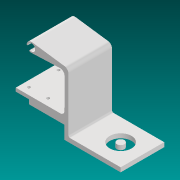
# Autodesk Inventor part: 链接板
Saved by Autodesk Inventor 2021 (Build 250183000, 183)
## iProperties
Created: 2025-04-17
Part Number: 链接板
Material: 常规
Document SubType Name: Modeling
Designer: 86155
Density: 1 g/cm^3
Appearance: 默认
Author: 86155
Autodesk Inventor part; units mm, degrees
ref_plane "YZ Plane" through (0, 0, 0) normal (1, 0, 0) x (0, 1, 0)
ref_plane "XZ Plane" through (0, 0, 0) normal (0, 1, 0) x (-1, 0, 0)
ref_plane "XY Plane" through (0, 0, 0) normal (0, 0, 1) x (1, 0, 0)
sketch "草图1" plane through (0, 0, 0) normal (0, 0, 1) x (1, 0, 0)
  circle A0 centre (0, 41) radius 4.25 projected
  circle A1 centre (0, 41) radius 4.25
  line L0 (0, 41) -> (-2.75, 36.2369)
  line L1 (0, 41) -> (5.5, 41) construction
  line L2 (0, 41) -> (-5.5, 41)
  line L3 (0.7501, 46.4486) -> (42.3728, 40.7189)
  line L4 (-15, 3) -> (-15, 6) projected
  line L5 (-15, 6) -> (-18, 6) projected
  line L6 (-18, 6) -> (-18, -8) projected
  line L7 (-4, -8) -> (-18, -8) projected
  line L8 (-4, -6) -> (-4, -8) projected
  line L9 (-4, -6) -> (4, -6) projected
  line L10 (4, -6) -> (4, -8) projected
  line L11 (18, -8) -> (4, -8) projected
  line L12 (18, 6) -> (18, -8) projected
  line L13 (18, 6) -> (15, 6) projected
  line L14 (15, 6) -> (15, 3) projected
  line L15 (15, 3) -> (13.5, 3) projected
  line L16 (13.5, 3) -> (13.5, 2) projected
  line L17 (13.5, 2) -> (15, 2) projected
  line L18 (15, 2) -> (15, -2) projected
  line L19 (15, -2) -> (-15, -2) projected
  line L20 (-15, -2) -> (-15, 2) projected
  line L21 (-15, 2) -> (-13.5, 2) projected
  line L22 (-13.5, 2) -> (-13.5, 3) projected
  line L23 (-13.5, 3) -> (-15, 3) projected
  line L24 (-18, -8) -> (18, -8)
  line L25 (18, -8) -> (18, -12)
  line L26 (18, -12) -> (-18, -12)
  line L27 (-18, -12) -> (-18, -8)
  line L28 (18, -12) -> (42.3728, -12)
  line L29 (42.3728, -12) -> (42.3728, 40.7189)
  line L30 (18, -8) -> (38, -8)
  line L31 (38, -8) -> (38, 37.0777)
  line L32 (0.2288, 35.5048) -> (38, 37.0777)
  arc A2 (-2.75, 36.2369) -> (0.2288, 35.5048) centre (0, 41) ccw
  arc A3 (0.7501, 46.4486) -> (-5.5, 41) centre (0, 41) ccw
  point P0 (0, 0)
  point P1 (-4.25, 41)
  point P2 (-2.125, 37.3194)
  dimension "d1" = 120
  dimension "d2" = 4
  dimension "d3" = 20
  constraints: 26 end point, 4 horizontal, 4 point on circle, 3 centre point, 3 perpendicular, 2 coincident, 2 parallel, 2 tangent, 1 concentric, 1 equal length, 1 point on line
  measures "d1" angle of L0 L1
  measures "d2" distance of L24.end L25.end
  measures "d3" distance of L24.end L30.end
extrude "拉伸1" add sketch "草图1" against normal blind 50 contours A0 L2 A3 L3 L29 L28 L25 L30 L31 L32 A2 L0 | L26 L27 L7 L24 L11 L25
fillet "圆角1" radius 5 2 edges at (38, 37.0777, -25) (42.3728, 40.7189, -25)
fillet "圆角2" radius 5 2 edges at (38, -8, -25) (42.3728, -12, -25)
sketch "草图2" plane through (-18, -12, -50) normal (0, -1, 0) x (1, 0, 0)
  line L0 (0, 50) -> (55.3728, 50) projected
  line L1 (0, 50) -> (0, 0) projected
  line L2 (55.3728, 0) -> (0, 0) projected
  point P0 (18, 50)
  point P1 (7, 42)
  point P2 (7, 8)
  point P3 (29, 42)
  point P4 (29, 8)
  dimension "d8" = 8
  dimension "d9" = 7
  dimension "d10" = 8
  dimension "d11" = 22
  measures "d8" distance from line of L0 point (7, 42)
  measures "d9" distance from line of L1 point (7, 42)
  measures "d10" distance from line of L2 point (7, 8)
  measures "d11" distance of point (29, 42) point (7, 42)
hole "孔1" at (-11, -12, -8) at (-11, -12, -42) at (11, -12, -8) at (11, -12, -42) direction (0, 1, 0) diameter 3.242 depth 4 tip angle 118 countersink diameter 4 countersink angle 90 thread size "M4x0.7" designation "M4" class "6H" standard "GB Metric profile"
sketch "草图5" plane through (0, 0, 0) normal (0, 0, 1) x (1, 0, 0)
  line L0 (42.3728, 36.36) -> (42.3728, -7) projected
  line L1 (42.3728, 0) -> (37.8728, 0)
  line L2 (37.8728, 0) -> (37.8728, -32)
  line L3 (37.8728, -32) -> (42.3728, -32)
  line L4 (42.3728, -32) -> (42.3728, 0)
  line L5 (37.8728, -32) -> (102.3728, -32)
  line L6 (102.3728, -32) -> (102.3728, -27)
  line L7 (102.3728, -27) -> (37.8728, -27)
  line L8 (37.8728, -27) -> (37.8728, -32)
  point P0 (0, 0)
  point P1 (42.3728, -27)
  dimension "d26" = 4.5
  dimension "d27" = 32
  dimension "d28" = 64.5
  dimension "d29" = 5
  constraints: 16 end point, 4 parallel, 2 horizontal, 2 perpendicular, 1 point on line
  measures "d26" distance of L3.end L2.end
  measures "d27" distance of L2.end L1.end
  measures "d28" distance of L7.end L6.end
  measures "d29" distance between parallel lines of L5 L7
extrude "拉伸4" add sketch "草图5" against normal blind 50
fillet "圆角3" radius 2 1 edges at (42.3728, -27, -25)
sketch "草图6" plane through (37.8728, -32, 0) normal (0, -1, 0) x (1, 0, 0)
  circle A0 centre (39.5, -25) radius 4.25 projected
  circle A1 centre (39.5, -25) radius 12.5
  point P0 (-37.8728, 0)
  dimension "d33" = 25
  constraints: 1 centre point, 1 coincident
  measures "d33" diameter of A1
extrude "拉伸5" cut sketch "草图6" against normal blind 10
sketch "草图7" plane through (-18, -12, -50) normal (0, -1, 0) x (1, 0, 0)
  line L0 (0, 50) -> (0, 0) projected
  line L1 (55.8728, 0) -> (55.8728, 50) projected
  line L2 (0, 35) -> (55.8728, 35)
  line L3 (55.8728, 35) -> (55.8728, 15)
  line L4 (55.8728, 15) -> (0, 15)
  line L5 (0, 15) -> (0, 35)
  line L6 (0, 50) -> (55.3728, 50) projected
  point P0 (18, 50)
  point P1 (0, 15)
  dimension "d36" = 20
  dimension "d37" = 15
  constraints: 8 end point, 2 parallel, 2 point on line, 1 horizontal, 1 perpendicular
  measures "d36" distance between parallel lines of L4 L2
  measures "d37" distance between parallel lines of L6 L2
extrude "拉伸6" add sketch "草图7" along normal up to surface (20 mm away)
sketch "草图8" plane through (37.8728, -32, 0) normal (0, -1, 0) x (1, 0, 0)
  line L0 (-55.8728, -15) -> (0, -15) projected
  line L1 (-55.8728, -35) -> (-55.8728, -15) projected
  point P0 (-37.8728, 0)
  point P1 (-45.8728, -25)
  point P2 (-15.8728, -25)
  dimension "d40" = 10
  dimension "d41" = 10
  dimension "d42" = 30
  measures "d40" distance from line of L0 point (-45.873, -25)
  measures "d41" distance from line of L1 point (-45.873, -25)
  measures "d42" distance of point (-45.873, -25) point (-15.873, -25)
hole "孔2" at (-8, -32, -25) at (22, -32, -25) direction (0, 1, 0) diameter 6.647 depth 18 thread size "M8x1.25" designation "M8" class "6H" standard "GB Metric profile"
